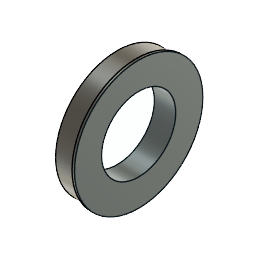
CrankShaft & bushing (Autodesk Fusion 360 design; units mm, degrees)
part number: 2026-05-15-13-15-11-933
Autodesk Fusion 360 part; units mm, degrees
sketch "Sketch1" plane through (0, 0, 0) normal (1, 0, 0) x (0, 1, 0)
  circle A0 centre (0, 0) radius 63.5
  circle A1 centre (0, 0) radius 38.1
  dimension "d1" = 127
  dimension "d2" = 76.2
  constraint coincident A0.centre A1.centre
  constraint concentric A0 A1
  measures "d1" diameter of A0
  measures "d2" diameter of A1
extrude "Extrude1" add sketch "Sketch1" along normal blind 19.5
sketch "Sketch2" plane through (19.5, 0, 0) normal (1, 0, 0) x (0, 1, 0)
  circle A0 centre (0, 0) radius 38.1
  circle A1 centre (0, 0) radius 63.5
  circle A2 centre (0, 0) radius 66.04
  dimension "d5" = 2.54
extrude "Extrude2" add sketch "Sketch2" along normal blind 2.54 contours A1 | A2
sketch "Sketch3" plane through (22.04, 0, 0) normal (1, 0, 0) x (0, 1, 0)
  circle A0 centre (0, 0) radius 38.1
  circle A1 centre (0, 0) radius 66.04
